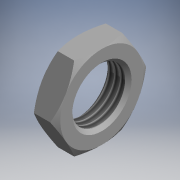
# Autodesk Inventor part: 10-CJ210Z_NUT
Saved by Autodesk Inventor 2017.3 (Build 213256000, 256)
## iProperties
Part Number: 10-CJ210Z_NUT
Material: Generic
Catalog Web Link: www.cadenas.de
Description: 10/11-CJ2-Z_NUT-Air Cylinder/Standard: Double Acting Single Rod/Clean Series
Vendor: SMC
Document SubType Name: Modeling
Designer: partserver
Manufacturer: SMC
Mass: 0.414663 g
Surface Area: 4.87707 cm^2
Volume: 0.414663 cm^3
Density: 1 g/cm^3
Appearance: PSOLRGB-191-191-191
Category: PARTsolutions
Company: SMC
Title: 10-CJ210Z_NUT
Author: Cadenas PARTsolutions
Comments: Air Cylinder/Standard: Double Acting Single Rod/Clean Series
PSOL_IDENT_0: {$CADENAS_DATA\23d-libs\smc_jp\actuator\standard_air_cylinder\cj2\10_cj2_z\parts\10_cj2_z_nut.prj},1
PSOL_IDENT_1: 75 {VTYP=3D},{NB=10-CJ210Z_NUT},{LINA=10-CJ210Z_NUT},{NN=10/11-CJ2-Z_NUT},{DATE=29.10.2021 06:22:38}
PSOL_IDENT_2: ,{GEOMDATE=08.07.2016 03:22:39},{VERSION=},{LINEID=10},{WBVAR=},{WBNUMERIC=}  {NB=10-CJ210Z_NUT},{LI
PSOL_IDENT_3: NA=10-CJ210Z_NUT},{KT=DUMMY},{BORE=10.000},{NN=M10x1},{NNA=10.000},{NNP=1.000},{H=14.000},{D=4.000}
NB: 10-CJ210Z_NUT
NN: M10x1
NT: Air Cylinder/Standard: Double Acting Single Rod/Clean Series
NBSYN: 10-CJ2$BORE.Z_NUT
LINA: 10-CJ210Z_NUT
CATALOG: SMC (JP
BORE: 10
NNA: 10
NNP: 1
H: 14
D: 4
SUPPLIER: SMC
ARTICLENO: 10-CJ210Z_NUT
BOMINFO: 10-CJ210Z_NUT
CREATOR: CADENAS GmbH
Autodesk Inventor part; units mm, degrees
sketch "Sketch_1" plane through (0, 0, 0) normal (0, 0, 1) x (1, 0, 0)
  line L0 (50, 0) -> (-50, 0)
  line L1 (0, 7) -> (0, 5)
  line L2 (0, 5) -> (0.5415, 4.4585)
  line L3 (0.5415, 4.4585) -> (3.4585, 4.4585)
  line L4 (3.4585, 4.4585) -> (4, 5)
  line L5 (4, 5) -> (4, 7)
  line L6 (4, 7) -> (2.3834, 9.8)
  line L7 (2.3834, 9.8) -> (1.6166, 9.8)
  line L8 (1.6166, 9.8) -> (0, 7)
  constraints: 18 end point
revolve "Revolution1" add sketch "Sketch_1" angle 360 about axis through (50, 0, 0) along (1, 0, 0)
thread "Thread1" size "M10x1" class "6H" standard "ISO Metric profile" full length
sketch "Sketch_2" plane through (0, 0, 0) normal (1, 0, 0) x (0, 1, 0)
  circle A0 centre (0, 0) radius 14
  line L0 (-4.0415, 7) -> (-8.0829, 0)
  line L1 (-8.0829, 0) -> (-4.0415, -7)
  line L2 (-4.0415, -7) -> (4.0415, -7)
  line L3 (4.0415, -7) -> (8.0829, 0)
  line L4 (8.0829, 0) -> (4.0415, 7)
  line L5 (4.0415, 7) -> (-4.0415, 7)
  constraints: 12 end point, 1 centre point
extrude "Extrusion1" cut sketch "Sketch_2" along normal blind 4
ref_plane "NUT_XY" through (0, 0, 0) normal (1, 0, 0) x (0, 0, -1)
ref_plane "NUT_YZ" through (0, 0, 0) normal (0, 0, -1) x (0, 1, 0)
ref_plane "NUT_ZX" through (0, 0, 0) normal (0, 1, 0) x (1, 0, 0)
body "Solid1"
